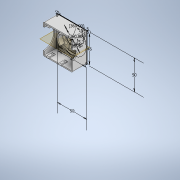
# Autodesk Inventor part: magnet_chargeBase_v2
Saved by Autodesk Inventor 2022 (Build 260153000, 153)
## iProperties
Created: 2022-07-31
Part Number: magnet_chargeBase_v2
Material: Generic
Document SubType Name: Modeling
Designer: sgioj
Density: 1 g/cm^3
Appearance: Default
Author: sgioj
Autodesk Inventor part; units mm, degrees
ref_plane "YZ Plane" through (0, 0, 0) normal (1, 0, 0) x (0, 1, 0)
ref_plane "XZ Plane" through (0, 0, 0) normal (0, 1, 0) x (-1, 0, 0)
ref_plane "XY Plane" through (0, 0, 0) normal (0, 0, 1) x (1, 0, 0)
sketch "Sketch1" plane through (0, 0, 0) normal (0, 0, 1) x (1, 0, 0)
  line L0 (0, 0) -> (50, 0)
  line L1 (50, 0) -> (50, -50)
  line L2 (50, -50) -> (0, -50)
  line L3 (0, -50) -> (0, 0)
  line L4 (2, -2) -> (48, -2)
  line L5 (48, -2) -> (48, -48)
  line L6 (48, -48) -> (2, -48)
  line L7 (2, -48) -> (2, -2)
  line L8 (2, -2) -> (48, -48) construction
  line L9 (48, -2) -> (2, -48) construction
  circle A0 centre (25, -25) radius 19.375
  circle A1 centre (25, -25) radius 14.5
  circle A2 centre (25, -25) radius 4.175
  circle A3 centre (31.678, -18.322) radius 2.65
  circle A4 centre (25, -15.5559) radius 2.65
  circle A5 centre (18.322, -18.322) radius 2.65
  circle A6 centre (15.5559, -25) radius 2.65
  circle A7 centre (18.322, -31.678) radius 2.65
  circle A8 centre (25, -34.4441) radius 2.65
  circle A9 centre (31.678, -31.678) radius 2.65
  circle A10 centre (34.4441, -25) radius 2.65
  line L10 (50, -25) -> (-10.9328, -25) construction
  line L11 (47.5, -2.5) -> (47.5, -17.5)
  line L12 (47.5, -2.5) -> (32.5, -2.5)
  line L13 (32.5, -2.5) -> (47.5, -17.5)
  line L14 (2.5, -17.5) -> (17.5, -2.5)
  line L15 (2.5, -2.5) -> (17.5, -2.5)
  line L16 (2.5, -2.5) -> (2.5, -17.5)
  line L17 (17.5, -47.5) -> (2.5, -32.5)
  line L18 (2.5, -47.5) -> (2.5, -32.5)
  line L19 (2.5, -47.5) -> (17.5, -47.5)
  line L20 (47.5, -32.5) -> (32.5, -47.5)
  line L21 (47.5, -47.5) -> (32.5, -47.5)
  line L22 (47.5, -47.5) -> (47.5, -32.5)
  line L23 (33.5518, -16.4482) -> (35.253, -14.747)
  line L24 (33.5518, -33.5518) -> (35.253, -35.253)
  arc A11 (16.4482, -16.4482) -> (16.4487, -33.5524) centre (24.9958, -25) ccw
  line L25 (16.4482, -16.4482) -> (14.747, -14.747)
  line L26 (16.4487, -33.5524) -> (14.747, -35.253)
  dimension "d7" = 5.3
  dimension "d0" = 50
  dimension "d1" = 50
  dimension "d2" = 46
  dimension "d3" = 46
  dimension "d4" = 38.75
  dimension "d5" = 29
  dimension "d6" = 8.35
  dimension "d10" = 360
  dimension "d12" = 2
  dimension "d13" = 2
  dimension "d49" = 15
  dimension "d50" = 15
  dimension "d51" = 2.5
  dimension "d52" = 2.5
  dimension "d55" = 360
  constraints: 54 end point, 9 point on line, 8 centre point, 6 point on circle, 4 horizontal, 4 parallel, 3 coincident, 3 midpoint, 2 perpendicular, 1 vertical, 55 other
  measures "d0" distance of L1.end L2.end
  measures "d1" distance of L0.end L1.end
  measures "d2" distance of L5.end L6.end
  measures "d3" distance of L4.end L5.end
  measures "d4" diameter of A0
  measures "d5" diameter of A1
  measures "d6" diameter of A2
  measures "d12" distance between parallel lines of L3 L7
  measures "d13" distance between parallel lines of L0 L4
  measures "d49" distance of L11.start L11.end
  measures "d50" distance of L11.start L12.end
  measures "d51" horizontal distance of L11.start L0.end
  measures "d52" distance from line of L1 L11.start
extrude "Extrusion1" add sketch "Sketch1" along normal blind 4 contours L4 L5 L6 L7 | A1 L26 A11 L25 | L25 A11 L26 A1 | L11 L13 L12 | L16 L15 L14 | L19 L18 L17 | L22 L21 L20
extrude "Extrusion2" add sketch "Sketch1" along normal blind 24 contours L0 L1 L2 L3
extrude "Extrusion3" add sketch "Sketch1" against normal blind 1 contours L0 L1 L2 L3 | L4 L5 L6 L7 | A0 | A5 | A6 | A7 | A1 L26 A11 L25 | L25 A11 L26 A1 | A2 | A3 | A4 | A8 | A9 | A10 | L11 L13 L12 | L16 L15 L14 | L19 L18 L17 | L22 L21 L20
sketch "Sketch2" plane through (2, -48, 4) normal (0, 1, 0) x (1, 0, 0)
  line L0 (46, -20) -> (0, -20) projected
  line L1 (5, -20) -> (9, -20)
  line L2 (9, -20) -> (9, -10)
  line L3 (9, -10) -> (5, -10)
  line L4 (5, -10) -> (5, -20)
  line L5 (0, 0) -> (0, -20) projected
  point P0 (-2, 4)
  dimension "d20" = 4
  dimension "d21" = 10
  dimension "d39" = 5
  constraints: 8 end point, 2 parallel, 1 horizontal, 1 perpendicular, 1 point on line
  measures "d20" distance of L3.end L2.end
  measures "d21" distance of L2.end L1.end
  measures "d39" distance between parallel lines of L4 L5
extrude "Extrusion4" add sketch "Sketch2" along normal blind 1.85
sketch "Sketch3" plane through (11, -48, 24) normal (1, 0, 0) x (0, 0, -1)
  line L0 (0, 1.85) -> (10, 1.85) projected
  line L1 (10, 0) -> (0, 0) projected
  line L2 (0, 1.85) -> (8, 1.85)
  line L3 (8, 1.85) -> (8, 0)
  line L4 (8, 0) -> (0, 0)
  line L5 (0, 0) -> (0, 1.85)
  line L6 (8, 1.85) -> (6.7272, 0.5772)
  line L7 (8, 1.85) -> (9.8, 1.85) construction
  line L8 (6.7272, 0.5772) -> (5.4544, 1.85)
  point P0 (24, 48)
  dimension "d24" = 8
  dimension "d25" = 1.8
  dimension "d26" = 135
  dimension "d27" = 1.8
  constraints: 14 end point, 2 horizontal, 2 parallel, 2 point on line, 1 equal length, 1 perpendicular
  measures "d24" distance of L3.end L4.end
  measures "d25" distance of L2.end L6.end
  measures "d26" angle of L6 L7
  measures "d27" distance of L6.end L8.end
extrude "Extrusion5" cut sketch "Sketch3" against normal blind 4 contours L0 L6 L8
sketch "Sketch4" plane through (2, -46.15, 4) normal (0, 1, 0) x (1, 0, 0)
  point P0 (-2, 4)
chamfer "Chamfer1" distance 1.5 angle 45 1 edges at (9, -46.15, 14)
sketch "Sketch5" plane through (0, -50, 24) normal (-1, 0, 0) x (0, 0, 1)
  line L0 (0, 50) -> (0, 0) projected
  circle A0 centre (0, 25) radius 17.5
  point P0 (-24, 50)
  point P1 (0, 7.5)
  point P2 (0, 42.5)
  dimension "d33" = 35
  constraints: 1 centre point, 1 midpoint
  measures "d33" diameter of A0
extrude "Extrusion6" cut sketch "Sketch5" against normal blind 2 contours L0 A0 picked at (-8.1651, 27.7367)
sketch "Sketch6" plane through (50, -50, 24) normal (1, 0, 0) x (0, 0, -1)
  line L0 (0, 0) -> (0, 50) projected
  circle A0 centre (0, 25) radius 7.5
  point P0 (24, 50)
  point P1 (0, 32.5)
  point P2 (0, 17.5)
  dimension "d36" = 15
  constraints: 1 centre point, 1 midpoint
  measures "d36" diameter of A0
extrude "Extrusion7" cut sketch "Sketch6" against normal blind 2 contours L0 A0 picked at (3.0672, 26.5587)
sketch "Sketch7" plane through (0, 0, 24) normal (0, 0, 1) x (1, 0, 0)
  line L0 (7, -47.4228) -> (7, -46.15) projected
  line L1 (11, -47.8) -> (7, -47.8)
  line L2 (7, -47.8) -> (7, -46.15)
  line L3 (7, -46.15) -> (11, -46.15)
  line L4 (11, -46.15) -> (11, -47.8)
  point P0 (0, 0)
  constraints: 8 end point, 2 parallel, 1 horizontal, 1 perpendicular
extrude "Extrusion8" add sketch "Sketch7" along normal blind 2
chamfer "Chamfer2" distance 1.5 angle 45 1 edges at (9, -46.15, 26)
pattern_linear "Rectangular Pattern1" count 2 spacing 21 along (1, 0, 0) of "Extrusion4", "Chamfer1", "Extrusion5", "Extrusion8", "Chamfer2"
ref_plane "Work Plane1" through (50, -25, 0) normal (0, 1, 0) x (-1, 0, 0)
mirror "Mirror1" about plane through (50, -25, 0) normal (0, 1, 0) of "Extrusion4", "Chamfer1", "Extrusion5", "Extrusion8", "Chamfer2", "Rectangular Pattern1"
extrude "Extrusion9" cut sketch "Sketch1" along normal blind 4 contours L11 L13 L12 | L16 L15 L14 | L19 L18 L17 | L22 L21 L20
fillet "Fillet1" radius 2 8 edges at (25, 0, -1) (0, -25, -1) (25, -50, -1) (50, -25, -1) (0, -50, 11.5) (0, 0, 11.5) (50, 0, 11.5) (50, -50, 11.5)
extrude "Extrusion10" add sketch "Sketch1" along normal blind 10.9 contours L25 A11 L26 A1 picked at (14.1377, -16.7711)
body "Solid1"
